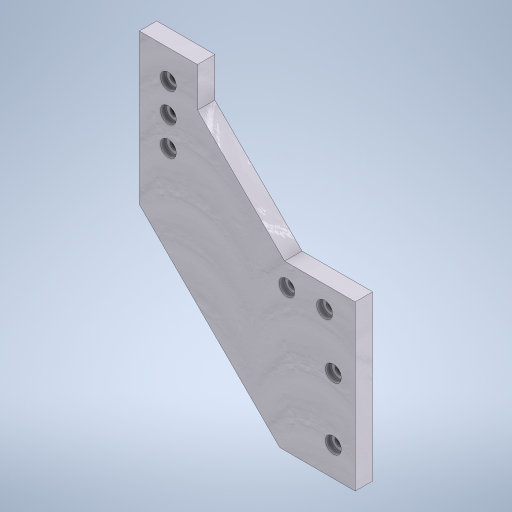
# Autodesk Inventor part: Plate_standard_low_3D
Saved by Autodesk Inventor 2023 (Build 270158000, 158)
## iProperties
Created: 2024-02-04
Part Number: Plate_standard_low_3D
Material: Aluminum 6061, Welded
Document SubType Name: Modeling
Designer: victo
Density: 2.7 g/cm^3
Appearance: Weld - Aluminum
Author: victo
Autodesk Inventor part; units mm, degrees
ref_plane "YZ Plane" through (0, 0, 0) normal (1, 0, 0) x (0, 1, 0)
ref_plane "XZ Plane" through (0, 0, 0) normal (0, 1, 0) x (-1, 0, 0)
ref_plane "XY Plane" through (0, 0, 0) normal (0, 0, 1) x (1, 0, 0)
sketch "Sketch1" plane through (0, 0, 0) normal (0, 0, 1) x (1, 0, 0)
  line L0 (0, 0) -> (-78.3, 0)
  line L1 (-78.3, 0) -> (-78.3, 100)
  line L2 (-78.3, 100) -> (0, 100)
  line L3 (0, 100) -> (0, 0)
  circle A0 centre (-11.5, 10) radius 1.5
  circle A1 centre (-11.5, 31.4) radius 1.5
  circle A2 centre (-14.5, 48.9) radius 1.5
  circle A3 centre (-27.5, 48.9) radius 1.5
  circle A4 centre (-68.3, 90) radius 1.5
  circle A5 centre (-68.3, 80) radius 1.5
  circle A6 centre (-68.3, 70) radius 1.5
  line L4 (0, 56.4) -> (-28.3, 56.4)
  line L5 (-28.3, 56.4) -> (-58.3, 86.4)
  line L6 (-58.3, 86.4) -> (-58.3, 100)
  line L7 (-30, 0) -> (-78.3, 48.3)
  dimension "d0" = 100
  dimension "d1" = 78.3
  dimension "d2" = 3
  dimension "d3" = 3
  dimension "d4" = 3
  dimension "d5" = 3
  dimension "d6" = 3
  dimension "d7" = 3
  dimension "d8" = 3
  dimension "d9" = 10
  dimension "d10" = 10
  dimension "d11" = 10
  dimension "d12" = 10
  dimension "d13" = 10
  dimension "d14" = 10
  dimension "d15" = 11.5
  dimension "d16" = 10
  dimension "d17" = 11.5
  dimension "d18" = 14.5
  dimension "d19" = 21.4
  dimension "d23" = 28.3
  dimension "d24" = 135
  dimension "d25" = 135
  dimension "d26" = 48.3
  dimension "d27" = 56.4
  dimension "d28" = 20
  dimension "d31" = 13
  dimension "d32" = 17.5
  dimension "d45" = 17.5
  constraints: 16 end point, 7 centre point, 4 point on line, 2 horizontal, 2 parallel, 2 perpendicular
  measures "d0" distance of L0.end L1.end
  measures "d1" distance between parallel lines of L3 L1
  measures "d2" diameter of A0
  measures "d3" diameter of A1
  measures "d4" diameter of A2
  measures "d5" diameter of A3
  measures "d6" diameter of A4
  measures "d7" diameter of A5
  measures "d8" diameter of A6
  measures "d9" distance from line of L2 A4.centre
  measures "d10" distance from line of L1 A4.centre
  measures "d11" distance from line of L1 A5.centre
  measures "d12" distance from line of L1 A6.centre
  measures "d13" distance of A4.centre A5.centre
  measures "d14" distance of A5.centre A6.centre
  measures "d15" distance from line of L3 A0.centre
  measures "d16" distance from line of L0 A0.centre
  measures "d17" distance from line of L3 A1.centre
  measures "d18" distance from line of L3 A2.centre
  measures "d19" distance of A1.centre A0.centre
  measures "d23" distance of L4.start L4.end
  measures "d24" angle of L4 L5
  measures "d25" angle of L0 L7
  measures "d26" distance of L0.end L7.start
  measures "d27" distance between parallel lines of L0 L4
  measures "d28" distance between parallel lines of L1 L6
  measures "d31" distance of A3.centre A2.centre
  measures "d32" vertical distance of A1.centre A3.centre
  measures "d45" vertical distance of A1.centre A2.centre
extrude "Extrusion1" add sketch "Sketch1" along normal blind 6 contours L0 L7 L1 L2 L6 L5 L4 L3
sketch "Sketch2" plane through (0, 0, 6) normal (0, 0, 1) x (1, 0, 0)
  line L0 (-30, 0) -> (0, 0) projected
  line L1 (0, 56.4) -> (-28.3, 56.4) projected
  line L2 (0, 0) -> (-4, 0)
  line L3 (-4, 0) -> (-4, 56.4)
  line L4 (-4, 56.4) -> (0, 56.4)
  line L5 (0, 56.4) -> (0, 0)
  dimension "d33" = 4
  constraints: 8 end point, 2 parallel, 1 horizontal, 1 perpendicular, 1 point on line
  measures "d33" distance of L3.end L4.end
extrude "Extrusion2" cut sketch "Sketch2" against normal blind 6
sketch "Sketch3" plane through (0, 0, 6) normal (0, 0, 1) x (1, 0, 0)
  circle A0 centre (-11.5, 10) radius 1.5 projected
  circle A1 centre (-11.5, 31.4) radius 1.5 projected
  circle A2 centre (-11.5, 10) radius 2.75
  circle A3 centre (-11.5, 31.4) radius 1.5 projected
  circle A4 centre (-11.5, 31.4) radius 2.75
  circle A5 centre (-14.5, 48.9) radius 1.5 projected
  circle A6 centre (-27.5, 48.9) radius 1.5 projected
  circle A7 centre (-68.3, 70) radius 1.5 projected
  circle A8 centre (-68.3, 80) radius 1.5 projected
  circle A9 centre (-68.3, 90) radius 1.5 projected
  circle A10 centre (-14.5, 48.9) radius 1.5 projected
  circle A11 centre (-14.5, 48.9) radius 2.75
  circle A12 centre (-27.5, 48.9) radius 1.5 projected
  circle A13 centre (-27.5, 48.9) radius 2.75
  circle A14 centre (-68.3, 70) radius 1.5 projected
  circle A15 centre (-68.3, 70) radius 2.75
  circle A16 centre (-68.3, 80) radius 1.5 projected
  circle A17 centre (-68.3, 80) radius 2.75
  circle A18 centre (-68.3, 90) radius 1.5 projected
  circle A19 centre (-68.3, 90) radius 2.75
  point P0 (0, 0)
  dimension "d36" = 5.5
  dimension "d37" = 5.5
  dimension "d40" = 5.5
  dimension "d41" = 5.5
  dimension "d42" = 5.5
  dimension "d43" = 5.5
  dimension "d44" = 5.5
  constraints: 7 centre point, 7 coincident
  measures "d36" diameter of A2
  measures "d37" diameter of A4
  measures "d40" diameter of A11
  measures "d41" diameter of A13
  measures "d42" diameter of A15
  measures "d43" diameter of A17
  measures "d44" diameter of A19
extrude "Extrusion3" cut sketch "Sketch3" against normal blind 2 contours A0 | A1 | A2 | A4 | A5 | A6 | A7 | A8 | A9 | A11 | A13 | A15 | A17 | A19
equation "\"d10\" = d9"
equation "\"d11\" = d9"
equation "\"d12\" = d11"
equation "\"d14\" = d13"
equation "\"d17\" = d15"
equation "\"d25\" = d24"
body "Solid1"
